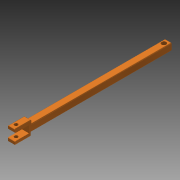
# Autodesk Inventor part: 2
Saved by Autodesk Inventor 2015 (Build 190159000, 159)
## iProperties
Created: 2016-03-11
Part Number: 2
Material: Złote
Document SubType Name: Modeling
Designer: Arek
Density: 19.3 g/cm^3
Appearance: Gorący metal 1600F
Mass: 11329.6 g
Surface Area: 849.664 cm^2
Volume: 587.027 cm^3
Author: Arek
Autodesk Inventor part; units mm, degrees
ref_plane "YZ Plane" through (0, 0, 0) normal (1, 0, 0) x (0, 1, 0)
ref_plane "XY Plane" through (0, 0, 0) normal (0, 0, 1) x (1, 0, 0)
sketch "Szkic1" plane through (0, 0, 0) normal (0, 1, 0) x (-1, 0, 0)
  line L0 (15, 0) -> (-15, 0)
  line L1 (-15, 0) -> (-15, -600)
  line L2 (-15, -600) -> (15, -600)
  line L3 (15, -600) -> (15, 0)
  point P0 (0, 0)
  point P1 (0, 0)
  dimension "d0" = 30
  dimension "d1" = 600
  constraints: 8 end point, 2 coincident, 2 parallel, 1 horizontal, 1 midpoint, 1 perpendicular
  measures "d0" distance of L2.end L1.end
  measures "d1" distance of L1.end L0.end
extrude "Wyciągnięcie proste1" add sketch "Szkic1" along normal blind 30
sketch "Szkic2" plane through (-15, 0, 0) normal (0, 0, 1) x (1, 0, 0)
  line L0 (0, 0) -> (0, 30) projected
  line L1 (0, 0) -> (30, 0) projected
  line L2 (30, 0) -> (30, 30) projected
  line L3 (0, 30) -> (30, 30) projected
  line L4 (0, 0) -> (0, 30) projected
  line L5 (0, -15) -> (30, -15)
  line L6 (30, -15) -> (30, 45)
  line L7 (30, 45) -> (0, 45)
  line L8 (0, 45) -> (0, -15)
  point P0 (15, 0)
  point P1 (0, 15)
  point P2 (0, 15)
  dimension "d4" = 60
  dimension "d5" = 30
  constraints: 8 end point, 2 midpoint, 2 parallel, 1 coincident, 1 horizontal, 1 perpendicular
  measures "d4" distance between parallel lines of L7 L5
  measures "d5" distance between parallel lines of L6 L8
extrude "Wyciągnięcie proste2" add sketch "Szkic2" along normal blind 10
sketch "Szkic3" plane through (-15, 0, 10) normal (0, 0, 1) x (1, 0, 0)
  line L0 (0, -15) -> (30, -15) projected
  line L1 (30, -15) -> (30, 45) projected
  line L2 (0, -15) -> (30, -15)
  line L3 (30, -15) -> (30, 0)
  line L4 (30, 0) -> (0, 0)
  line L5 (0, 0) -> (0, -15)
  point P0 (15, 0)
  constraints: 8 end point, 2 parallel, 1 horizontal, 1 perpendicular, 1 point on line
extrude "Wyciągnięcie proste3" add sketch "Szkic3" along normal blind 60
ref_plane "Płaszczyzna konstrukcyjna1" through (0, 15, 0) normal (0, 1, 0) x (-1, 0, 0)
mirror "Odbicie lustrzane1" about plane through (0, 15, 0) normal (0, 1, 0) of "Wyciągnięcie proste3"
sketch "Szkic4" plane through (0, 15, 0) normal (0, 1, 0) x (-1, 0, 0)
  point P0 (0, 0)
sketch "Szkic5" plane through (-15, 45, 0) normal (0, 1, 0) x (1, 0, 0)
  line L0 (0, -70) -> (30, -70) projected
  line L1 (30, 0) -> (30, -70) projected
  circle A0 centre (15, -50) radius 7.5
  point P0 (15, 0)
  dimension "d11" = 15
  dimension "d12" = 20
  dimension "d13" = 15
  constraints: 1 centre point
  measures "d11" diameter of A0
  measures "d12" distance from line of A0.centre L0
  measures "d13" distance from line of L1 A0.centre
extrude "Wyciągnięcie proste4" cut sketch "Szkic5" against normal through all
fillet "Zaokrąglenie1" radius 4 12 edges at (0, 45, 0) (0, 45, 70) (0, 0, 70) (-15, 0, -300) (-15, 30, -300) (-15, 15, -600) (0, 0, -600) (0, 30, -600) (15, 15, -600) (15, 0, -300) (15, 30, -300) (0, -15, 0)
sketch "Szkic6" plane through (0, 0, 0) normal (0, -1, 0) x (1, 0, 0)
  circle A0 centre (0, -580) radius 10
  line L0 (-11, -600) -> (11, -600) projected
  line L1 (-15, 0) -> (-15, -596) projected
  point P0 (0, 0)
  dimension "d17" = 20
  dimension "d18" = 20
  dimension "d19" = 15
  constraints: 1 centre point
  measures "d17" diameter of A0
  measures "d18" distance from line of L0 A0.centre
  measures "d19" distance from line of L1 A0.centre
extrude "Wyciągnięcie proste5" cut sketch "Szkic6" against normal through all
fillet "Zaokrąglenie2" radius 4 3 edges at (0, -15, 70) (15, -3.5, 0) (-15, -3.5, 0)
fillet "Zaokrąglenie3" radius 4 1 edges at (0, 30, 70)
